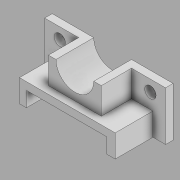
# Autodesk Inventor part: Pieza3
Saved by Autodesk Inventor 2020 (Build 240168000, 168)
## iProperties
Created: 2019-08-15
Part Number: Pieza3
Material: Genérico
Document SubType Name: Modeling
Designer: gerar
Density: 1 g/cm^3
Appearance: Valor por defecto
Author: gerar
Autodesk Inventor part; units mm, degrees
ref_plane "YZ Plane" through (0, 0, 0) normal (1, 0, 0) x (0, 1, 0)
ref_plane "XZ Plane" through (0, 0, 0) normal (0, 1, 0) x (-1, 0, 0)
ref_plane "XY Plane" through (0, 0, 0) normal (0, 0, 1) x (1, 0, 0)
sketch "Boceto1" plane through (0, 0, 0) normal (0, 0, 1) x (1, 0, 0)
  line L0 (0, 0) -> (152.4, 0)
  line L1 (152.4, 0) -> (152.4, 61.9125)
  line L2 (152.4, 61.9125) -> (0, 61.9125)
  line L3 (0, 61.9125) -> (0, 0)
  dimension "d0" = 152.4
  dimension "d1" = 61.9125
  constraints: 8 end point, 2 parallel, 1 horizontal, 1 perpendicular
  measures "d0" distance of L2.end L1.end
  measures "d1" distance of L1.end L0.end
extrude "Bloque_Posterior" add sketch "Boceto1" along normal blind 9.525
sketch "Boceto2" plane through (0, 0, 9.525) normal (0, 0, 1) x (1, 0, 0)
  line L0 (15.875, 0) -> (136.525, 0)
  line L1 (136.525, 0) -> (136.525, 28.575)
  line L2 (136.525, 28.575) -> (15.875, 28.575)
  line L3 (15.875, 28.575) -> (15.875, 0)
  line L4 (0, 0) -> (152.4, 0) projected
  line L5 (76.2, 0) -> (76.2, 70.6909) construction
  dimension "d4" = 120.65
  dimension "d5" = 28.575
  dimension "d6" = 60.325
  constraints: 10 end point, 2 parallel, 1 horizontal, 1 midpoint, 1 perpendicular, 1 vertical
  measures "d4" distance of L2.end L1.end
  measures "d5" distance of L1.end L0.end
  measures "d6" distance between parallel lines of L5 L1
extrude "Bloque_Inferior" add sketch "Boceto2" along normal blind 47.625
sketch "Boceto3" plane through (0, 0, 9.525) normal (0, 0, 1) x (1, 0, 0)
  line L0 (0, 0) -> (152.4, 0) projected
  line L1 (76.2, 0) -> (76.2, 86.7708) construction
  line L2 (42.8625, 61.9125) -> (109.5375, 61.9125)
  line L3 (109.5375, 61.9125) -> (109.5375, 28.575)
  line L4 (109.5375, 28.575) -> (42.8625, 28.575)
  line L5 (42.8625, 28.575) -> (42.8625, 61.9125)
  line L6 (152.4, 61.9125) -> (0, 61.9125) projected
  dimension "d9" = 66.675
  dimension "d10" = 33.3375
  dimension "d11" = 33.3375
  constraints: 10 end point, 2 parallel, 1 collinear, 1 horizontal, 1 midpoint, 1 perpendicular, 1 vertical
  measures "d9" distance of L3.end L4.end
  measures "d10" distance of L2.end L3.end
  measures "d11" distance between parallel lines of L1 L3
extrude "Bloque_Superior" add sketch "Boceto3" along normal blind 38.1
sketch "Boceto4" plane through (0, 0, 9.525) normal (0, 0, 1) x (1, 0, 0)
  line L0 (0, 0) -> (152.4, 0) projected
  line L1 (24.5425, 0) -> (126.1425, 0)
  line L2 (126.1425, 0) -> (126.1425, 19.05)
  line L3 (126.1425, 19.05) -> (24.5425, 19.05)
  line L4 (24.5425, 19.05) -> (24.5425, 0)
  dimension "d14" = 101.6
  dimension "d15" = 19.05
  constraints: 8 end point, 2 parallel, 1 horizontal, 1 perpendicular, 1 point on line
  measures "d14" distance of L3.end L2.end
  measures "d15" distance of L2.end L1.end
extrude "Orificio_Inferior" cut sketch "Boceto4" along normal blind 47.625 and the other way blind 23.8252
sketch "Boceto5" plane through (0, 0, 47.625) normal (0, 0, 1) x (1, 0, 0)
  line L0 (109.5375, 61.9125) -> (42.8625, 61.9125) projected
  arc A0 (52.3875, 61.9125) -> (100.0125, 61.9125) centre (76.2, 61.9125) ccw
  point P0 (0, 0)
  dimension "d20" = 47.625
  constraints: 2 point on circle, 2 point on line, 1 centre point, 1 midpoint
  measures "d20" diameter of A0
extrude "Agujero_Central" cut sketch "Boceto5" against normal blind 47.625
sketch "Boceto6" plane through (0, 0, 9.525) normal (0, 0, 1) x (1, 0, 0)
  line L0 (-22.923, 47.625) -> (163.4069, 47.625) construction
  line L1 (19.05, -6.8102) -> (19.05, 78.4252) construction
  line L2 (42.8625, 61.9125) -> (0, 61.9125) projected
  line L3 (0, 61.9125) -> (0, 0) projected
  circle A0 centre (19.05, 47.625) radius 7.1437
  dimension "d23" = 14.2875
  dimension "d24" = 19.05
  dimension "d25" = 14.2875
  constraints: 4 end point, 2 point on line, 1 centre point, 1 horizontal, 1 vertical
  measures "d23" distance between parallel lines of L0 L2
  measures "d24" distance between parallel lines of L1 L3
  measures "d25" diameter of A0
extrude "Agujero_Izquierdo" cut sketch "Boceto6" against normal blind 9.525
sketch "Boceto7" plane through (0, 0, 9.525) normal (0, 0, 1) x (1, 0, 0)
  line L0 (133.35, 81.3516) -> (133.35, -20.5289) construction
  line L1 (173.8284, 47.625) -> (-5.5853, 47.625) construction
  line L2 (152.4, 0) -> (152.4, 61.9125) projected
  line L3 (152.4, 61.9125) -> (109.5375, 61.9125) projected
  circle A0 centre (133.35, 47.625) radius 7.1438
  point P0 (0, 0)
  dimension "d28" = 19.05
  dimension "d29" = 14.2875
  dimension "d30" = 14.2875
  constraints: 4 end point, 2 point on line, 1 centre point, 1 horizontal, 1 vertical
  measures "d28" distance between parallel lines of L2 L0
  measures "d29" distance between parallel lines of L1 L3
  measures "d30" diameter of A0
extrude "Agujero_Derecho" cut sketch "Boceto7" against normal blind 9.525
